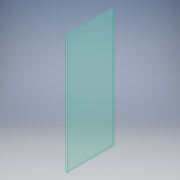
# Autodesk Inventor part: alas_komponen
Saved by Autodesk Inventor 2019 (Build 230136000, 136)
## iProperties
Created: 2020-07-18
Part Number: alas_komponen
Material: Generic
Document SubType Name: Modeling
Designer: Agus Prayudi
Density: 1 g/cm^3
Appearance: Indoor Pool
Author: Agus Prayudi
Autodesk Inventor part; units mm, degrees
ref_plane "YZ Plane" through (0, 0, 0) normal (1, 0, 0) x (0, 1, 0)
ref_plane "XZ Plane" through (0, 0, 0) normal (0, 1, 0) x (-1, 0, 0)
ref_plane "XY Plane" through (0, 0, 0) normal (0, 0, 1) x (1, 0, 0)
sketch "Sketch1" plane through (0, 0, 0) normal (0, 1, 0) x (-1, 0, 0)
  line L0 (-1, 41.328) -> (1, 41.328)
  line L1 (1, 41.328) -> (1, -41.328)
  line L2 (1, -41.328) -> (-1, -41.328)
  line L3 (-1, -41.328) -> (-1, 41.328)
  line L4 (-1, 41.328) -> (1, -41.328) construction
  line L5 (1, 41.328) -> (-1, -41.328) construction
  point P0 (0, 0)
  dimension "d0" = 2
  dimension "d1" = 82.656
  constraints: 12 end point, 2 midpoint, 2 parallel, 1 horizontal, 1 perpendicular
  measures "d0" distance of L1.end L2.end
  measures "d1" distance of L0.end L1.end
extrude "Extrusion1" add sketch "Sketch1" along normal blind 210
body "Solid1"
